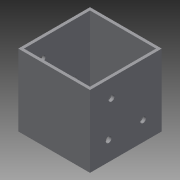
# Autodesk Inventor part: Arm_Parallel_Case
Saved by Autodesk Inventor 2013 (Build 170138000, 138)
## iProperties
Created: 2014-04-08
Part Number: Arm_Parallel_Case
Material: 一般
Document SubType Name: Modeling
Designer: andou
Density: 1 g/cm^3
Author: andou
Autodesk Inventor part; units mm, degrees
ref_plane "YZ Plane" through (0, 0, 0) normal (1, 0, 0) x (0, 1, 0)
ref_plane "XZ Plane" through (0, 0, 0) normal (0, 1, 0) x (-1, 0, 0)
ref_plane "XY Plane" through (0, 0, 0) normal (0, 0, 1) x (1, 0, 0)
sketch "スケッチ1" plane through (0, 0, 0) normal (0, 0, 1) x (1, 0, 0)
  line L0 (-25, 25) -> (25, 25)
  line L1 (25, 25) -> (25, -25)
  line L2 (25, -25) -> (-25, -25)
  line L3 (-25, -25) -> (-25, 25)
  line L4 (-23, 23) -> (23, 23)
  line L5 (23, 23) -> (23, -23)
  line L6 (23, -23) -> (-23, -23)
  line L7 (-23, -23) -> (-23, 23)
  point P0 (0, 0)
  dimension "d0" = 46
  dimension "d2" = 50
  dimension "d3" = 23
  dimension "d4" = 25
  dimension "d5" = 46
  dimension "d6" = 50
  dimension "d7" = 23
  dimension "d8" = 25
  constraints: 16 end point, 4 parallel, 2 horizontal, 2 perpendicular
  measures "d0" distance between parallel lines of L5 L7
  measures "d2" distance of L0.start L0.end
  measures "d3" distance from line of point (0, 0) L7
  measures "d4" distance from line of point (0, 0) L1
  measures "d5" distance between parallel lines of L6 L4
  measures "d6" distance between parallel lines of L0 L2
  measures "d7" distance from line of point (0, 0) L6
  measures "d8" distance from line of point (0, 0) L0
extrude "押し出し1" add sketch "スケッチ1" against normal blind 50
sketch "スケッチ2" plane through (25, -25, 0) normal (1, 0, 0) x (0, 0, -1)
  line L0 (0, 50) -> (0, 0) projected
  line L1 (0, 0) -> (50, 0) projected
  circle A0 centre (12.5, 15) radius 2
  circle A1 centre (36.5, 37) radius 2
  circle A2 centre (36.5, 13) radius 2
  point P0 (0, 25)
  dimension "d11" = 24
  dimension "d13" = 24
  dimension "d14" = 2
  dimension "d15" = 22
  dimension "d16" = 4
  dimension "d17" = 15
  dimension "d18" = 12.5
  constraints: 3 centre point, 2 equal radius
  measures "d11" horizontal distance of A2.centre A0.centre
  measures "d13" horizontal distance of A1.centre A0.centre
  measures "d14" vertical distance of A0.centre A2.centre
  measures "d15" vertical distance of A0.centre A1.centre
  measures "d16" diameter of A2
  measures "d17" distance from line of L1 A0.centre
  measures "d18" distance from line of A0.centre L0
hole "穴1" at (25, -10, -12.5) at (25, 12, -36.5) at (25, -12, -36.5) direction (-1, 0, 0) diameter 4 end through all
